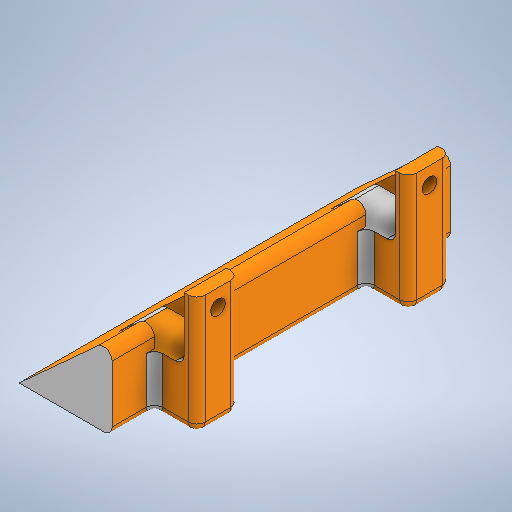
# Autodesk Inventor part: pare-chocs
Saved by Autodesk Inventor 2025 (Build 290162000, 162)
## iProperties
Created: 2024-10-10
Part Number: pare-chocs
Material: Générique
Document SubType Name: Modeling
Designer: chass
Density: 1 g/cm^3
Appearance: Par défaut
Author: chass
## iProperties of the stored document pare-chocs_Impression 3D.ipt
Created: 2025-01-09
Part Number: pare-chocs_Impression 3D
Material: Générique
Document SubType Name: Modeling
Designer: chass
Density: 1 g/cm^3
Appearance: Par défaut
Author: chass
Autodesk Inventor part; units mm, degrees
ref_plane "YZ Plane" through (0, 0, 0) normal (1, 0, 0) x (0, 1, 0)
ref_plane "XZ Plane" through (0, 0, 0) normal (0, 1, 0) x (-1, 0, 0)
ref_plane "XY Plane" through (0, 0, 0) normal (0, 0, 1) x (1, 0, 0)
sketch "Esquisse1" plane through (0, 0, 0) normal (1, 0, 0) x (0, 1, 0)
  line L0 (-2.5, 65) -> (2.5, 65)
  line L1 (2.5, 65) -> (2.5, -65)
  line L2 (2.5, -65) -> (-2.5, -65)
  line L3 (-2.5, -65) -> (-2.5, 65)
  line L4 (2.5, 65) -> (-2.5, -65)
  line L5 (2.5, -65) -> (-2.5, 65)
  point P0 (0, 0)
  point P1 (0, 0)
  point P2 (0, 0)
  dimension "d0" = 130
  dimension "d1" = 5
  constraints: 12 end point, 2 midpoint, 2 parallel, 1 coincident, 1 horizontal, 1 perpendicular
  measures "d0" distance of L0.end L1.end
  measures "d1" distance of L1.end L2.end
extrude "Extrusion1" add sketch "Esquisse1" along normal blind 5
sketch "Esquisse2" plane through (5, 0, 0) normal (1, 0, 0) x (0, 0, -1)
  line L0 (65, 2.5) -> (-65, 2.5) projected
  line L1 (-65, -2.5) -> (65, -2.5) projected
  line L2 (-30, 2.5) -> (-20, 2.5)
  line L3 (-20, 2.5) -> (-20, -2.5)
  line L4 (-20, -2.5) -> (-30, -2.5)
  line L5 (-30, -2.5) -> (-30, 2.5)
  line L6 (0, 13) -> (0, -16)
  line L7 (30, 2.5) -> (20, 2.5)
  line L8 (20, 2.5) -> (20, -2.5)
  line L9 (20, -2.5) -> (30, -2.5)
  line L10 (30, -2.5) -> (30, 2.5)
  point P0 (0, 0)
  point P1 (-20, 2.5)
  point P2 (30, -2.5)
  point P3 (30, 2.5)
  point P4 (20, 2.5)
  point P5 (20, -2.5)
  dimension "d4" = 10
  dimension "d5" = 20
  constraints: 18 end point, 4 symmetric about line, 3 point on line, 2 parallel, 1 horizontal, 1 perpendicular, 1 vertical
  measures "d4" distance between parallel lines of L3 L5
  measures "d5" distance between parallel lines of L3 L6
extrude "Extrusion2" add sketch "Esquisse2" along normal blind 10 contours L10 L1 L8 L0 | L3 L1 L5 L0
sketch "Esquisse3" plane through (0, 2.5, 65) normal (0, 1, 0) x (1, 0, 0)
  line L0 (15, 45) -> (15, 35) projected
  line L1 (5, 45) -> (15, 45) projected
  line L2 (15, 35) -> (12, 35)
  line L3 (12, 35) -> (12, 45)
  line L4 (12, 45) -> (15, 45)
  line L5 (15, 45) -> (15, 35)
  line L6 (-9, 65) -> (24, 65)
  line L7 (15, 85) -> (15, 95)
  line L8 (15, 95) -> (12, 95)
  line L9 (12, 95) -> (12, 85)
  line L10 (12, 85) -> (15, 85)
  line L11 (15, 85) -> (15, 95)
  point P0 (0, 65)
  constraints: 20 end point, 5 symmetric about line, 2 horizontal, 2 parallel, 1 perpendicular, 1 point on line
extrude "Extrusion3" add sketch "Esquisse3" along normal blind 15
sketch "Esquisse4" plane through (15, 0, 0) normal (1, 0, 0) x (0, 0, -1)
  circle A0 centre (-25, 13.5) radius 1.75
  line L0 (0, 20) -> (0, -21)
  circle A1 centre (25, 13.5) radius 1.75
  line L1 (-30, 17.5) -> (-20, 17.5) projected
  line L2 (-20, -2.5) -> (-20, 17.5) projected
  point P0 (0, 0)
  dimension "d10" = 3.5
  dimension "d11" = 4
  dimension "d19" = 5
  constraints: 2 centre point, 2 end point, 1 symmetric about line, 1 vertical, 1 other
  measures "d10" diameter of A0
  measures "d11" distance from line of L1 A0.centre
  measures "d19" distance from line of L2 A0.centre
extrude "Extrusion4" cut sketch "Esquisse4" against normal blind 10
sketch "Esquisse6" plane through (0, -2.5, 65) normal (0, 0, 1) x (1, 0, 0)
  line L0 (0, 0) -> (5, 0) projected
  line L1 (5, 0) -> (5, -8)
  line L2 (5, -8) -> (-17, -8)
  line L3 (-17, -8) -> (5, 12)
  line L4 (5, 0) -> (5, 5) projected
  line L5 (5, 12) -> (5, 0)
  point P0 (0, 2.5)
  constraints: 8 end point, 1 collinear, 1 perpendicular, 1 point on line, 1 vertical
extrude "Extrusion6" add sketch "Esquisse6" against normal blind 130
sketch "Esquisse8" plane through (12, 2.5, 20) normal (-1, 0, 0) x (0, 0, 1)
  line L0 (0, -5) -> (0, 15) projected
  line L1 (0, 0) -> (10, 0) projected
  line L2 (0, 15) -> (10, 15)
  line L3 (10, 15) -> (10, 0)
  line L4 (10, 0) -> (0, 0)
  line L5 (0, 0) -> (0, 15)
  line L6 (-50, -5) -> (-50, 15) projected
  line L7 (-40, 0) -> (-40, 15) projected
  line L8 (-50, 15) -> (-40, 15)
  line L9 (-40, 15) -> (-40, 0)
  line L10 (-40, 0) -> (-50, 0)
  line L11 (-50, 0) -> (-50, 15)
  circle A0 centre (5, 6) radius 1.75
  point P0 (-20, -2.5)
  constraints: 16 end point, 4 parallel, 2 horizontal, 2 perpendicular, 1 centre point, 1 coincident
extrude "Extrusion7" cut sketch "Esquisse8" along normal blind 130 contours L0 L2 L3 L1 | L6 L8 L7 L10 | A0
sketch "Esquisse10" plane through (5, -2.5, -30) normal (0, -1, 0) x (1, 0, 0)
  line L0 (10, 0) -> (7, 0) projected
  line L1 (0, 10) -> (7, 10) projected
  line L2 (10, 0) -> (0, 0)
  line L3 (0, 0) -> (0, 10)
  line L4 (0, 10) -> (10, 10)
  line L5 (10, 10) -> (10, 0)
  line L6 (0, 60) -> (7, 60) projected
  line L7 (10, 50) -> (0, 50)
  line L8 (0, 50) -> (0, 60)
  line L9 (0, 60) -> (10, 60)
  line L10 (10, 60) -> (10, 50)
  point P0 (-5, 30)
  constraints: 16 end point, 4 parallel, 2 horizontal, 2 perpendicular, 1 point on line
extrude "Extrusion8" add sketch "Esquisse10" along normal blind 8
fillet "Congé5" radius 2 20 edges at (15, -10.5, -25) (15, -10.5, 25) (5, -10.5, -47.5) (5, -10.5, 0) (5, -10.5, 47.5) (10, -10.5, 20) (10, -10.5, 30) (10, -10.5, -20) (10, -10.5, -30) (-6, -10.5, -65) (5, -0.5, -65) (-6, -0.5, -65) (5, 9.5, -47.5) (5, 9.5, 0) (5, 9.5, 47.5) (5, -0.5, 65) (15, 3.5, 30) (15, 3.5, 20) (15, 3.5, -20) (15, 3.5, -30)
fillet "Congé6" radius 2 10 edges at (8, -10.5, 28) (4.4142, -9.9142, 29.4142) (5, -3, 30) (4.4142, -9.9142, -20.5858) (5, -3, -20) (4.4142, -9.9142, 20.5858) (5, -3, 20) (8, -10.5, -28) (4.4142, -9.9142, -29.4142) (5, -3, -30)
fillet "Congé7" radius 2 2 edges at (12, 2.5, -25) (12, 2.5, 25)
fillet "Congé8" radius 2 2 edges at (-2.7, 2.5, -25) (-2.7, 2.5, 25)
sketch "Esquisse12" plane through (-17, -10.5, 65) normal (0, 0, 1) x (1, 0, 0)
  line L0 (0, 0) -> (22, 20)
  line L1 (22, 20) -> (22, 0)
  line L2 (22, 13) -> (22, 2) projected
  line L3 (22, 0) -> (0, 0)
  point P0 (17, 10.5)
  constraints: 6 end point, 1 collinear, 1 perpendicular, 1 point on line
extrude "Extrusion9" cut sketch "Esquisse12" against normal blind 25
sketch "Esquisse13" plane through (3, -8.5, -65) normal (0, 0, -1) x (-1, 0, 0)
  line L0 (0, -2) -> (20, -2) projected
  line L1 (20, -2) -> (-2, 18)
  line L2 (-2, 18) -> (-2, -2)
  line L3 (-2, 11) -> (-2, 0) projected
  line L4 (-2, -2) -> (20, -2)
  point P0 (3, 8.5)
  constraints: 6 end point, 1 collinear, 1 perpendicular
extrude "Extrusion10" cut sketch "Esquisse13" against normal blind 25
